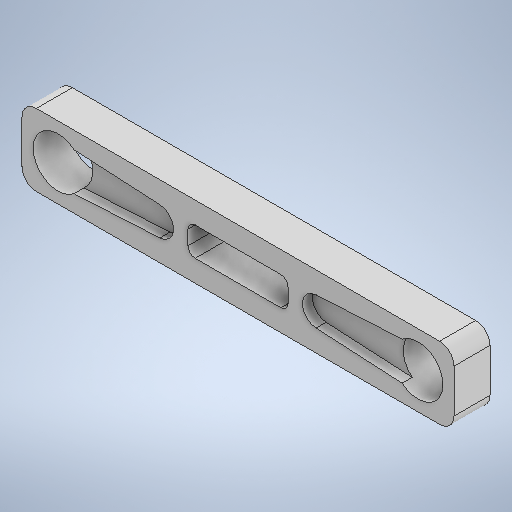
# Autodesk Inventor part: leg_v0.1
Saved by Autodesk Inventor 2025 (Build 290162000, 162)
## iProperties
Created: 2024-06-04
Part Number: leg_v0.1
Material: Generic
Document SubType Name: Modeling
Designer: sgols
Density: 1 g/cm^3
Appearance: Default
Mass: 1.31587 g
Surface Area: 16.6417 cm^2
Volume: 1.31587 cm^3
Author: sgols
Autodesk Inventor part; units mm, degrees
ref_plane "YZ Plane" through (0, 0, 0) normal (1, 0, 0) x (0, 1, 0)
ref_plane "XZ Plane" through (0, 0, 0) normal (0, 1, 0) x (-1, 0, 0)
sketch "Sketch1" plane through (0, 0, 0) normal (0, 0, 1) x (1, 0, 0)
  line L0 (0, 0) -> (60, 0)
  line L1 (60, 0) -> (60, 10)
  line L2 (60, 10) -> (0, 10)
  line L3 (0, 10) -> (0, 0)
  line L4 (30, 10) -> (30, 0) construction
  dimension "d0" = 60
  dimension "d2" = 10
  constraints: 10 end point, 2 midpoint, 2 parallel, 1 horizontal, 1 perpendicular
  measures "d0" distance of L0.start L0.end
  measures "d2" distance of L0.end L1.end
extrude "Extrusion1" add sketch "Sketch1" along normal mid plane 5
sketch "Sketch2" plane through (0, 0, 2.5) normal (0, 0, 1) x (1, 0, 0)
  circle A0 centre (5, 5) radius 3.45
  line L0 (60, 10) -> (0, 10) projected
  line L1 (60, 0) -> (60, 10) projected
  line L2 (60, 10) -> (0, 10) projected
  line L3 (0, 10) -> (0, 0) projected
  line L4 (0, 0) -> (60, 0) projected
  line L5 (7.2091, 7.65) -> (7.2091, 2.35) construction
  arc A1 (19.1591, 3.003) -> (19.1591, 6.997) centre (19.05, 5) ccw
  line L6 (7.2091, 7.65) -> (19.1591, 6.997)
  line L7 (5, 5) -> (19.05, 5) construction
  line L8 (7.2091, 2.35) -> (19.1591, 3.003)
  line L9 (0, 5) -> (5, 5) construction
  line L10 (5, 10) -> (5, 5) construction
  dimension "d8" = 6.9
  dimension "d9" = 5.3
  dimension "d10" = 14.05
  dimension "d11" = 2
  constraints: 12 end point, 4 point on circle, 2 centre point, 2 horizontal, 2 vertical, 1 horizontal alignment, 1 midpoint, 1 perpendicular, 1 point on line, 1 symmetric about line, 1 tangent
  measures "d8" diameter of A0
  measures "d9" distance of L5.start L5.end
  measures "d10" distance of L7.end L7.start
  measures "d11" radius of A1
extrude "Extrusion2" cut sketch "Sketch2" along normal through all both and the other way through all contours A0
extrude "Extrusion3" cut sketch "Sketch2" against normal blind 1.4 contours A0 L6 A1 L8
ref_plane "Work Plane1" through (30, 0, 2.5) normal (-1, 0, 0) x (0, 0, 1)
mirror "Mirror1" about plane through (30, 0, 2.5) normal (-1, 0, 0) of "Extrusion2", "Extrusion3"
fillet "Fillet1" radius 2 4 edges at (60, 10, 0) (60, 0, 0) (0, 0, 0) (0, 10, 0)
sketch "Sketch3" plane through (0, 0, 2.5) normal (0, 0, 1) x (1, 0, 0)
  line L0 (30, -2) -> (30, 12) projected
  line L1 (0, 8) -> (0, 2) projected
  line L2 (23.05, 7) -> (36.95, 7)
  line L3 (36.95, 7) -> (36.95, 3)
  line L4 (36.95, 3) -> (23.05, 3)
  line L5 (23.05, 3) -> (23.05, 7)
  line L6 (23.05, 7) -> (36.95, 3) construction
  line L7 (36.95, 7) -> (23.05, 3) construction
  arc A0 (40.8409, 6.997) -> (40.8409, 3.003) centre (40.95, 5) ccw construction
  line L8 (58, 10) -> (2, 10) construction
  line L9 (30, 7) -> (30, 10) construction
  line L10 (2, 0) -> (58, 0) projected
  point P0 (0, 0)
  point P1 (30, 5)
  point P2 (38.95, 5)
  point P3 (0, 5)
  dimension "d26" = 2
  dimension "d27" = 3
  constraints: 14 end point, 6 midpoint, 2 parallel, 1 horizontal, 1 horizontal alignment, 1 perpendicular, 1 point on circle
  measures "d26" distance from line of point (38.95, 5) L3
  measures "d27" distance between parallel lines of L8 L2
extrude "Extrusion4" cut sketch "Sketch3" against normal through all
fillet "Fillet2" radius 1 4 edges at (23.05, 7, 0) (23.05, 3, 0) (36.95, 3, 0) (36.95, 7, 0)
body "Solid1"
